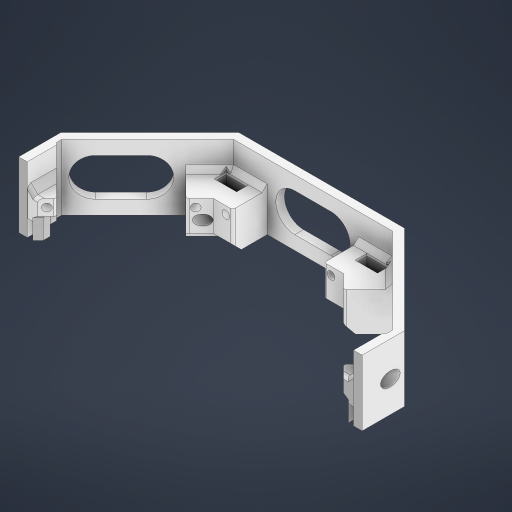
# Autodesk Inventor part: Držák TF-Luna
Saved by Autodesk Inventor 2024 (Build 280153000, 153)
## iProperties
Created: 2023-11-02
Part Number: Držák TF-Luna
Material: Všeobecné
Document SubType Name: Modeling
Designer: 42060
Density: 1 g/cm^3
Appearance: Výchozí
Author: 42060
Autodesk Inventor part; units mm, degrees
ref_plane "YZ Plane" through (0, 0, 0) normal (1, 0, 0) x (0, 1, 0)
ref_plane "XZ Plane" through (0, 0, 0) normal (0, 1, 0) x (-1, 0, 0)
ref_plane "XY Plane" through (0, 0, 0) normal (0, 0, 1) x (1, 0, 0)
sketch "Náčrt1" plane through (0, 0, 0) normal (0, 0, 1) x (1, 0, 0)
  line L0 (0, 0) -> (0, -2.5)
  line L1 (0, -2.5) -> (23, -2.5)
  line L2 (23, -2.5) -> (47.25, -26.75)
  line L3 (49.75, -25.714466) -> (24.035534, 0)
  line L4 (24.035534, 0) -> (0, 0)
  line L5 (49.75, -25.714466) -> (49.75, -37.923)
  line L6 (49.75, -37.923) -> (47.25, -37.923)
  line L7 (47.25, -37.923) -> (47.25, -26.75)
  dimension "d0" = 2.5
  dimension "d1" = 23
  dimension "d2" = 135
  dimension "d50" = 49.75
  dimension "d54" = 2.5
  dimension "d55" = 2.5
  dimension "d156" = 37.923
  constraints: 16 end point, 3 perpendicular, 2 vertical, 1 parallel
  measures "d0" distance of L0.start L0.end
  measures "d1" distance of L0.end L1.end
  measures "d2" angle of L2 L1
  measures "d50" distance between parallel lines of L5 L0
  measures "d54" distance between parallel lines of L2 L3
  measures "d55" distance between parallel lines of L5 L7
  measures "d156" distance between parallel lines of L6 L4
extrude "Vysunutí1" add sketch "Náčrt1" along normal mid plane 19
sketch "Náčrt2" plane through (0, -2.5, 9.5) normal (0, -1, 0) x (1, 0, 0)
  line L0 (23, -19) -> (23, 0) projected
  line L1 (0, 0) -> (23, 0) projected
  line L2 (0, -19) -> (0, 0) projected
  line L3 (23, -19) -> (0, -19) projected
  line L4 (13.25, -7.75) -> (15.25, -7.75)
  arc A0 (15.25, -12.25) -> (15.25, -7.75) centre (15.25, -10) ccw
  line L5 (15.25, -12.25) -> (13.25, -12.25)
  line L6 (13.25, -12.25) -> (13.25, -7.75)
  point P0 (0, -9.5)
  dimension "d6" = 2.25
  dimension "d8" = 9
  dimension "d148" = 13.25
  dimension "d149" = 15.25
  constraints: 6 end point, 2 point on circle, 2 tangent, 1 centre point, 1 horizontal, 1 parallel, 1 perpendicular
  measures "d6" radius of A0
  measures "d8" distance from line of L3 A0.centre
  measures "d148" distance between parallel lines of L6 L2
  measures "d149" distance from line of L2 A0.centre
extrude "Vysunutí2" add sketch "Náčrt2" along normal blind 10 contours L4 A0 L5 L6
sketch "Náčrt4" plane through (47.25, -26.75, 9.5) normal (-0.7071068, -0.7071068, 0) x (-0.7071068, 0.7071068, 0)
  line L0 (24.544679, 7.75) -> (26.544679, 7.75)
  arc A0 (26.544679, 7.75) -> (26.544679, 12.25) centre (26.544679, 10) ccw
  line L1 (26.544679, 12.25) -> (24.544679, 12.25)
  line L2 (24.544679, 12.25) -> (24.544679, 7.75)
  line L3 (0, 19) -> (0, 0)
  line L4 (34.294679, 0) -> (0, 0)
  line L5 (34.294679, 19) -> (34.294679, 0)
  line L6 (0, 19) -> (34.294679, 19)
  line L7 (41.18897, 12.25) -> (41.18897, 7.75)
  line L8 (11.294679, 19) -> (11.294679, 0) construction
  line L9 (-1.955321, 12.25) -> (-1.955321, 7.75)
  line L10 (-1.955321, 7.75) -> (-6.455321, 7.75)
  line L11 (-6.455321, 7.75) -> (-6.455321, 12.25)
  line L12 (-6.455321, 12.25) -> (-1.955321, 12.25)
  point P0 (52.325902, 9.5)
  point P1 (28.794679, 10)
  point P2 (-3.955321, 10)
  dimension "d22" = 15.25
  dimension "d33" = 2.25
  dimension "d39" = 5.5
  dimension "d150" = 13.25
  constraints: 16 end point, 4 perpendicular, 3 point on circle, 3 symmetric about line, 2 horizontal, 2 point on line, 2 tangent, 1 centre point, 1 horizontal alignment, 1 parallel, 1 vertical
  measures "d22" distance from line of L8 A0.centre
  measures "d33" radius of A0
  measures "d39" distance from line of L5 point (28.795, 10)
  measures "d150" distance between parallel lines of L8 L2
extrude "Vysunutí3" add sketch "Náčrt4" along normal blind 10 contours L2 L1 A0 L0 | L9 L10 L11 L12
sketch "Náčrt8" plane through (49.75, -37.923, 9.5) normal (1, 0, 0) x (0, 0, -1)
  line L0 (7.75, 8.673) -> (12.25, 8.673)
  line L1 (7.75, 6.608399) -> (7.75, 8.673)
  line L2 (12.25, 6.608399) -> (7.75, 6.608399)
  line L3 (12.25, 8.673) -> (12.25, 6.608399)
  line L4 (12.25, 4.543797) -> (7.75, 4.543797)
  line L5 (12.25, 6.608399) -> (12.25, 4.543797)
  line L6 (12.25, 6.608399) -> (7.75, 6.608399)
  line L7 (7.75, 6.608399) -> (7.75, 4.543797)
  point P0 (9.5, 37.923)
extrude "Vysunutí7" cut sketch "Náčrt8" along normal through all
sketch "Náčrt10" plane through (13.25, -2.5, 1.75) normal (0, 0, 1) x (1, 0, 0)
  line L0 (2, -10) -> (0, -10)
  line L1 (2, -10) -> (4.25, -10)
  line L2 (6.568019, -10.960155) -> (8.15901, -12.551145)
  line L3 (9.573223, -13.965359) -> (8.15901, -12.551145)
  line L4 (4.25, -10) -> (5.607864, -10)
  line L5 (5.607864, -10) -> (6.568019, -10.960155)
  circle A0 centre (7.844431, -4.600449) radius 3.594431
  line L6 (4.25, 0) -> (4.25, -10)
  line L7 (13.639087, -3.889087) -> (6.568019, -10.960155)
  line L8 (4.25, -4.600449) -> (2, -4.600449)
  line L9 (2, 0) -> (2, -10)
  line L10 (10.386078, -7.142096) -> (11.977069, -8.733087)
  line L11 (15.230078, -5.480078) -> (8.15901, -12.551145)
  line L12 (5.607864, -10) -> (6.468902, -7.921271) construction
  line L13 (-13.25, 0) -> (9.75, 0)
  line L14 (9.75, 0) -> (34, -24.25)
  point P0 (-13.25, 2.5)
  dimension "d70" = 112.5
  constraints: 10 end point, 4 point on line, 3 point on circle, 2 horizontal, 2 tangent, 1 centre point, 1 collinear, 1 equal length, 1 perpendicular
  measures "d70" angle of L4 L12
extrude "Vysunutí9" add sketch "Náčrt10" against normal up to surface (4.5 mm away) contours L9 L8 L6 L1 | L6 A0 L7 L5 L4 | L9 L13 L6 L8 | L7 L10 L11 L2 | L7 L14 L11 L10
sketch "Náčrt6" plane through (47.25, -26.75, 9.5) normal (-0.7071068, -0.7071068, 0) x (-0.7071068, 0.7071068, 0)
  arc A0 (11.391901, 8.259484) -> (11.391901, 10.740516) centre (16.544679, 9.5) ccw
  arc A1 (11.197457, 10.740516) -> (11.197457, 8.259484) centre (6.044679, 9.5) ccw
  line L0 (0, 19) -> (0, 0)
  line L1 (24.544679, 12.25) -> (24.544679, 7.75)
  line L2 (-1.955321, 7.75) -> (-1.955321, 12.25)
  line L3 (16.544679, 9.5) -> (24.544679, 9.5) construction
  line L4 (6.044679, 9.5) -> (-1.955321, 9.5) construction
  arc A2 (11.391901, 8.259484) -> (11.197457, 8.259484) centre (11.294679, 8.236078) ccw
  arc A3 (11.197457, 10.740516) -> (11.391901, 10.740516) centre (11.294679, 10.763922) ccw
  arc A4 (11.294679, 7.86064) -> (11.294679, 11.13936) centre (16.544679, 9.5) ccw
  arc A5 (11.294679, 11.13936) -> (11.294679, 7.86064) centre (6.044679, 9.5) ccw
  line L5 (16.544679, 4) -> (6.044679, 4)
  line L6 (16.544679, 15) -> (6.044679, 15)
  point P0 (52.325902, 9.5)
  point P1 (12.501786, 10.226292)
  point P2 (12.501786, 8.773708)
  point P3 (0, 9.5)
  point P4 (12.599008, 10.740516)
  point P5 (12.404563, 10.740516)
  point P6 (12.404563, 8.259484)
  point P7 (12.599008, 8.259484)
  dimension "d44" = 10.6
  dimension "d45" = 10.5
  dimension "d48" = 0.2
  dimension "d114" = 0.2
  constraints: 16 point on circle, 8 end point, 7 tangent, 6 centre point, 3 point on line, 2 equal radius, 2 horizontal alignment, 1 collinear, 1 midpoint, 1 parallel, 1 perpendicular, 1 other
  measures "d44" diameter of A1
  measures "d45" distance of L4.start L3.start
  measures "d48" diameter of A2
  measures "d114" radial gap between concentric circles of A0 A4
extrude "Vysunutí5" cut sketch "Náčrt6" against normal blind 11.5 contours A2 A1 A3 A0 | A5 A4 | A4 L5 A5 | A4 A5 L6
sketch "Náčrt7" plane through (0, -2.5, 9.5) normal (0, -1, 0) x (1, 0, 0)
  arc A0 (0.097222, -10.740516) -> (0.097222, -8.259484) centre (5.25, -9.5) ccw
  line L0 (0, -19) -> (0, 0)
  arc A1 (0, -8.336078) -> (0.097222, -8.259484) centre (0, -8.236078) ccw
  arc A2 (0.097222, -10.740516) -> (0, -10.663922) centre (0, -10.763922) ccw
  arc A3 (-0.097222, -8.259484) -> (-0.097222, -10.740516) centre (-5.25, -9.5) ccw
  arc A4 (-0.097222, -8.259484) -> (0, -8.336078) centre (0, -8.236078) ccw
  arc A5 (0, -10.663922) -> (-0.097222, -10.740516) centre (0, -10.763922) ccw
  arc A6 (0, -7.86064) -> (0, -11.13936) centre (-5.25, -9.5) ccw
  arc A7 (0, -11.13936) -> (0, -7.86064) centre (5.25, -9.5) ccw
  line L1 (-5.25, -4) -> (5.25, -4)
  line L2 (-5.25, -15) -> (5.25, -15)
  point P0 (0, -9.5)
  point P1 (0, -9.5)
  point P2 (0, -8.773708)
  point P3 (0, -10.226292)
  point P4 (0, -9.5)
  point P5 (0.097222, -8.259484)
  point P6 (0, -8.336078)
  point P7 (0, -10.663922)
  point P8 (0.097222, -10.740516)
  point P9 (0, -8.136078)
  point P10 (0, -10.863922)
  point P11 (0, -11.13936)
  point P12 (0, -15)
  point P13 (0, -4)
  dimension "d40" = 10.6
  dimension "d41" = 5.25
  dimension "d49" = 0.2
  dimension "d115" = 0.2
  constraints: 20 point on circle, 8 centre point, 6 tangent, 4 end point, 3 symmetric about line, 2 midpoint, 2 point on line, 2 vertical alignment, 1 equal radius, 1 horizontal alignment, 4 other
  measures "d40" diameter of A0
  measures "d41" distance from line of A0.centre L0
  measures "d49" diameter of A1
  measures "d115" radial gap between concentric circles of A3 A6
extrude "Vysunutí4" cut sketch "Náčrt7" against normal blind 11.5 contours A2 L0 A1 A0 | A0 A1 L0 A7 A2 | A5 A3 A4 L0 | A7 L2 L0 | L0 L1 A7
sketch "Náčrt11" plane through (0, 0, -9.5) normal (0, 0, -1) x (-1, 0, 0)
  line L0 (-23, -2.5) -> (0, -2.5)
  line L1 (-47.25, -26.75) -> (-23, -2.5)
  line L2 (-13.25, -2.5) -> (-13.25, -12.5)
  line L3 (-13.25, -12.5) -> (-18.857864, -12.5)
  line L4 (-18.857864, -12.5) -> (-22.823223, -16.465359)
  line L5 (-29.894291, -9.394291) -> (-22.823223, -16.465359)
  arc A0 (-23.636078, -9.642096) -> (-17.5, -7.100449) centre (-21.094431, -7.100449) ccw
  line L6 (-17.5, -7.100449) -> (-17.5, -2.5)
  line L7 (-26.889087, -6.389087) -> (-23.636078, -9.642096)
  point P0 (0, 0)
extrude "Vysunutí10" add sketch "Náčrt11" against normal up to surface (6.75 mm away) contours L0 L2 L3 L4 L5 L1 L7 A0 L6
sketch "Náčrt3" plane through (0, -12.5, 9.5) normal (0, -1, 0) x (1, 0, 0)
  arc A0 (15.25, -12.25) -> (15.25, -7.75) centre (15.25, -10) ccw projected
  point P0 (0, -9.5)
  constraints: 1 coincident
hole "Díra1" at (15.25, -12.5, -0.5) direction (0, 1, 0) diameter 2.2 end through all
sketch "Náčrt5" plane through (40.178932, -33.821068, 9.5) normal (-0.7071068, -0.7071068, 0) x (0, 0, -1)
  arc A0 (7.75, -26.544679) -> (12.25, -26.544679) centre (10, -26.544679) ccw
  line L0 (12.25, 6.455321) -> (7.75, 6.455321)
  line L1 (7.75, 6.455321) -> (7.75, 1.955321)
  line L2 (7.75, 1.955321) -> (12.25, 1.955321)
  line L3 (12.25, 1.955321) -> (12.25, 6.455321)
  line L4 (12.25, 1.955321) -> (12.25, 6.455321)
  line L5 (12.25, 6.455321) -> (7.75, 6.455321)
  line L6 (19, 1.035534) -> (0, 1.035534)
  line L7 (0, 9.668271) -> (0, 1.035534)
  line L8 (19, 9.668271) -> (0, 9.668271)
  line L9 (19, 1.035534) -> (19, 9.668271)
  line L10 (19, -11.294679) -> (0, -11.294679) construction
  point P0 (9.5, -52.325902)
  point P1 (10, 3.955321)
  constraints: 1 coincident, 1 symmetric about line
hole "Díra2" at (21.40901, -15.051145, -0.5) at (42.975767, -36.617902, -0.5) direction (0.7071068, 0.7071068, 0) diameter 2.2 end through all
chamfer "Zkosení3" [suppressed]
sketch "Náčrt9" plane through (47.25, -35.879203, 1.75) normal (0, 0, 1) x (1, 0, 0)
  line L0 (0, -2.043797) -> (0, 9.129203)
  line L1 (0, 0) -> (-2.506466, -2.506466)
  line L2 (0, -2.043797) -> (-2.043797, -2.043797)
  line L3 (-2.043797, -2.043797) -> (-2.969136, -2.043797)
  line L4 (-2.506466, -2.506466) -> (-5.688447, 0.675514)
  line L5 (0, 9.129203) -> (0, -2.043797)
  point P0 (-47.25, 35.879203)
  constraints: 4 end point, 2 horizontal, 2 point on line
extrude "Vysunutí8" add sketch "Náčrt9" against normal up to surface (4.5 mm away) contours L2 L1 L0
extrude "Vysunutí17" cut sketch "Náčrt9" against normal through all contours L1 L4 L3
sketch "Náčrt25" plane through (47.25, -35.879203, -2.75) normal (0, 0, -1) x (-1, 0, 0)
  line L0 (1.5, 2.956203) -> (1.5, -2.043797)
  line L1 (1.5, -2.043797) -> (3, -0.543797)
  line L2 (3, -0.543797) -> (3, 1.456203)
  line L3 (3, 1.456203) -> (1.5, 2.956203)
  line L4 (0, -2.043797) -> (0, 9.129203)
  point P0 (47.25, 35.879203)
  dimension "d185" = 45
  dimension "d188" = 1.5
  dimension "d189" = 5
  dimension "d190" = 1.5
  dimension "d191" = 45
  constraints: 8 end point, 1 horizontal alignment, 1 parallel, 1 vertical
  measures "d185" angle of L3 L0
  measures "d188" distance between parallel lines of L0 L2
  measures "d189" distance of L0.start L0.end
  measures "d190" distance between parallel lines of L4 L0
  measures "d191" angle of L0 L1
extrude "Vysunutí24" add sketch "Náčrt25" along normal up to surface (6.75 mm away)
chamfer "Zkosení4" [suppressed]
chamfer "Zkosení10" distance 2 angle 45 2 edges at (47.25, -33.7191, 1.75) (47.25, -33.7191, -2.75)
chamfer "Zkosení11" distance 1.0388 angle 45 3 edges at (44.75, -33.923, -2.75) (44.25, -35.423, -2.75) (44.75, -36.923, -2.75)
sketch "Náčrt26" plane through (47.25, -37.923, 9.5) normal (0, -1, 0) x (1, 0, 0)
  line L0 (0, -14.25) -> (-1.5, -14.25)
  line L1 (2.5, -19) -> (2.5, 0)
  line L2 (0, 0) -> (2.5, 0)
  line L3 (0, -5.75) -> (0, 0)
  line L4 (-2, -7.75) -> (0, -5.75)
  line L5 (-2.969136, -7.75) -> (-2, -7.75)
  line L6 (-2.969136, -12.25) -> (-2.969136, -7.75)
  line L7 (-2.969085, -12.25) -> (-2.969136, -12.25)
  line L8 (-2.969085, -12.25) -> (-1.5, -13.2888)
  line L9 (-1.5, -12.75) -> (-1.5, -13.2888)
  line L10 (0, -14.25) -> (-1.5, -12.75)
  line L11 (0, -19) -> (0, -14.25)
  line L12 (2.5, -19) -> (0, -19)
  line L13 (-1.5, -13.2888) -> (-1.5, -19)
  point P0 (-47.25, -9.5)
  constraints: 2 end point, 1 horizontal
extrude "Vysunutí25" add sketch "Náčrt26" against normal up to surface contours L0 L13 L9 L10 surface through (44.25, -34.423, -2.75) normal (-0.7071068, 0.7071068, 0)
extrude "Vysunutí21" add sketch "Náčrt11" against normal blind 2.5 contours L0 L6 A0 L7 L1
sketch "Náčrt22" plane through (17.5, -2.5, -7) normal (0, 0, 1) x (1, 0, 0)
  line L0 (0, -1.850449) -> (5.8, -1.850449)
  line L1 (5.8, -1.850449) -> (5.8, -4.600449)
  line L2 (5.8, -4.600449) -> (0, -4.600449)
  line L3 (0, -4.600449) -> (0, -1.850449)
  line L4 (0, -4.600449) -> (0, 0)
  arc A0 (0, -4.600449) -> (6.136078, -7.142096) centre (3.594431, -4.600449) ccw
  line L5 (9.389087, -3.889087) -> (6.136078, -7.142096)
  line L6 (5.5, 0) -> (9.389087, -3.889087)
  line L7 (0, 0) -> (5.5, 0)
  point P0 (-17.5, 2.5)
  point P1 (0, -1.850449)
  dimension "d163" = 5.8
  dimension "d164" = 2.75
  constraints: 8 end point, 2 parallel, 1 collinear, 1 horizontal, 1 perpendicular, 1 point on line
  measures "d163" distance of L1.end L2.end
  measures "d164" distance of L0.end L1.end
extrude "Vysunutí20" add sketch "Náčrt22" along normal up to surface (8.75 mm away) contours L4 L7 L6 L5 A0 L2 L1 L0
sketch "Náčrt23" plane through (17.5, -4.350449, -7) normal (0, -1, 0) x (1, 0, 0)
  line L0 (5.8, 8.75) -> (0, 8.75)
  line L1 (0, 0) -> (0, 8.75)
  line L2 (5.8, 0) -> (0, 0)
  line L3 (5.8, 0) -> (5.8, 8.75)
  line L4 (0, 1.674316) -> (2.9, 0)
  line L5 (2.9, 0) -> (5.8, 1.674316)
  circle A0 centre (2.9, 3.348632) radius 2.9 construction
  point P0 (-17.5, 7)
  dimension "d169" = 120
  constraints: 4 end point, 3 tangent, 2 point on line, 1 centre point, 1 horizontal alignment, 1 midpoint
  measures "d169" angle of L5 L4
extrude "Vysunutí22" add sketch "Náčrt23" along normal up to surface (2.75 mm away) contours L3 L2 L5 | L4 L2 L1
hole "Díra6" at (20.4, -4.350449, -3.651368) direction (0, 1, 0) diameter 3 end through all both
sketch "Náčrt24" plane through (0, 0, -9.5) normal (0, 0, -1) x (-1, 0, 0)
  line L0 (0, 0) -> (-24.035534, 0)
  line L1 (-21.9, 0) -> (-18.9, 0)
  line L2 (-18.9, -4.350449) -> (-21.9, -4.350449)
  line L3 (-24.491911, -3) -> (-16.308089, -3)
  line L4 (-24.491911, -3) -> (-23.4, 0)
  line L5 (-16.308089, -3) -> (-17.4, 0)
  point P0 (-20.4, -3)
  point P1 (-20.4, -4.350449)
  dimension "d180" = 3
  dimension "d183" = 70
  dimension "d184" = 70
  dimension "d209" = 6
  constraints: 6 end point, 2 midpoint, 2 point on line, 1 vertical alignment
  measures "d180" distance between parallel lines of L0 L3
  measures "d183" angle of L0 L4
  measures "d184" angle of L0 L5
  measures "d209" distance of L4.end L5.end
extrude "Vysunutí23" cut sketch "Náčrt24" against normal blind 10
fillet "Zaoblení1" radius 1 2 edges at (46.25, -37.923, 2.75) (44.7654, -37.923, 1.75)
chamfer "Zkosení5" distance 1.5 angle 45 2 edges at (26.4471, -5.9471, 1.75) (18.125, -2.5, 1.75)
sketch "Náčrt12" plane through (0, 0, 9.5) normal (0, 1, 0) x (1, 0, 0)
  circle A0 centre (15.25, 10) radius 1.1
  line L0 (15.25, 12.424871) -> (17.35, 11.212436)
  line L1 (17.35, 11.212436) -> (17.35, 8.787564)
  line L2 (17.35, 8.787564) -> (15.25, 7.575129)
  line L3 (15.25, 7.575129) -> (13.15, 8.787564)
  line L4 (13.15, 8.787564) -> (13.15, 11.212436)
  line L5 (13.15, 11.212436) -> (15.25, 12.424871)
  point P0 (0, 9.5)
  point P1 (15.25, 10)
  dimension "d81" = 4.2
  constraints: 12 end point, 1 coincident, 1 vertical alignment, 13 other
  measures "d81" distance between parallel lines of L4 L1
extrude "Vysunutí12" [suppressed]
sketch "Náčrt13" plane through (24.035534, 0, -9.5) normal (0.7071068, 0.7071068, 0) x (-0.7071068, 0.7071068, 0)
  circle A0 centre (-8.785534, 9) radius 1.1
  line L0 (-8.785534, 6.575129) -> (-10.885534, 7.787564)
  line L1 (-10.885534, 7.787564) -> (-10.885534, 10.212436)
  line L2 (-10.885534, 10.212436) -> (-8.785534, 11.424871)
  line L3 (-8.785534, 11.424871) -> (-6.685534, 10.212436)
  line L4 (-6.685534, 10.212436) -> (-6.685534, 7.787564)
  line L5 (-6.685534, 7.787564) -> (-8.785534, 6.575129)
  line L6 (-39.285534, 6.575129) -> (-41.385534, 7.787564)
  line L7 (-41.385534, 7.787564) -> (-41.385534, 10.212436)
  line L8 (-41.385534, 10.212436) -> (-39.285534, 11.424871)
  line L9 (-39.285534, 11.424871) -> (-37.185534, 10.212436)
  line L10 (-37.185534, 10.212436) -> (-37.185534, 7.787564)
  line L11 (-37.185534, 7.787564) -> (-39.285534, 6.575129)
  circle A1 centre (-39.285534, 9) radius 1.1
  point P0 (16.995689, 9.5)
  point P1 (-39.285534, 9)
  point P2 (-39.285534, 9)
  dimension "d84" = 4.2
  dimension "d85" = 4.2
  constraints: 24 end point, 3 coincident, 1 vertical alignment, 26 other
  measures "d84" distance between parallel lines of L4 L1
  measures "d85" distance between parallel lines of L7 L10
extrude "Vysunutí13" [suppressed]
extrude "Vysunutí14" [suppressed]
sketch "Náčrt15" plane through (0, 0, 9.5) normal (0, 1, 0) x (1, 0, 0)
  circle A0 centre (15.25, 10) radius 1.1 projected
  point P0 (0, 9.5)
  point P1 (15.25, 10)
  constraints: 1 coincident
hole "Díra3" at (15.25, 0, -0.5) direction (0, -1, 0) diameter 4 depth 2
sketch "Náčrt16" plane through (24.035534, 0, -9.5) normal (0.7071068, 0.7071068, 0) x (-0.7071068, 0.7071068, 0)
  circle A0 centre (-8.785534, 9) radius 1.1
  point P0 (16.995689, 9.5)
  constraints: 1 coincident
hole "Díra4" at (30.247845, -6.212311, -0.5) direction (-0.7071068, -0.7071068, 0) diameter 4 depth 2
sketch "Náčrt17" plane through (24.035534, 0, -9.5) normal (0.7071068, 0.7071068, 0) x (-0.7071068, 0.7071068, 0)
  circle A0 centre (-39.285534, 9) radius 1.1
  point P0 (16.995689, 9.5)
  point P1 (-39.285534, 9)
  point P2 (-39.285534, 9)
  constraints: 2 coincident
hole "Díra5" at (51.814601, -27.779067, -0.5) direction (-0.7071068, -0.7071068, 0) diameter 4 depth 6
sketch "Náčrt14" plane through (49.75, -37.923, 9.5) normal (1, 0, 0) x (0, 0, -1)
  line L0 (19, 12.208534) -> (0, 12.208534)
  line L1 (19, 12.208534) -> (23, 12.208534)
  line L2 (23, 12.208534) -> (23, 6.208534)
  line L3 (23, 6.208534) -> (21, 6.208534)
  line L4 (21, 6.208534) -> (21, 10.208534)
  line L5 (21, 10.208534) -> (19, 10.208534)
  line L6 (19, 12.208534) -> (19, 0)
  point P0 (9.5, 37.923)
  point P1 (11.381206, 11.708534)
  dimension "d105" = 2
  dimension "d106" = 2
  dimension "d107" = 6
  dimension "d108" = 4
  constraints: 10 end point, 3 perpendicular, 1 horizontal, 1 vertical, 1 other
  measures "d105" distance between parallel lines of L1 L5
  measures "d106" distance between parallel lines of L4 L2
  measures "d107" distance between parallel lines of L1 L3
  measures "d108" distance between parallel lines of L6 L2
extrude "Vysunutí15" [suppressed]
chamfer "Zkosení7" [suppressed]
chamfer "Zkosení1" distance 2.5 angle 45 2 edges at (16.0539, -12.5, -9.5) (20.8405, -14.4827, -9.5)
fillet "Zaoblení3" radius 0.7 3 edges at (13.25, -12.5, -2.625) (22.8232, -16.4654, -2.625) (41.5616, -35.2037, -0.5)
sketch "Náčrt19" plane through (49.75, -37.923, 9.5) normal (1, 0, 0) x (0, 0, -1)
  line L0 (0, 11.173) -> (0, 0) projected
  line L1 (0, 0) -> (19, 0)
  line L2 (19, 0) -> (19, -0.077)
  line L3 (19, -0.077) -> (0, -0.077)
  line L4 (0, -0.077) -> (0, 0)
  point P0 (9.5, 37.923)
  dimension "d153" = 38
  constraints: 8 end point, 2 parallel, 1 horizontal, 1 perpendicular
  measures "d153" distance from line of point (9.5, 37.923) L3
extrude "Vysunutí18" add sketch "Náčrt19" against normal up to surface (2.5 mm away)
sketch "Náčrt20" plane through (0, 0, 9.5) normal (0, 0, 1) x (1, 0, 0)
  line L0 (23, -2.5) -> (47.25, -26.75)
  line L1 (47.25, -26.75) -> (48.632621, -28.132621)
  line L2 (48.632621, -28.132621) -> (47.25, -29.515242)
  line L3 (47.25, -26.75) -> (47.25, -38)
  line L4 (47.882621, -27.382621) -> (47.882621, -28.882621)
  line L5 (45.25, -31.515242) -> (42.056528, -34.708714)
  point P0 (0, 0)
  dimension "d159" = 0.75
  constraints: 6 end point, 4 point on line, 1 collinear, 1 perpendicular, 1 vertical
  measures "d159" distance from line of L1.end L4
extrude "Vysunutí19" cut sketch "Náčrt20" against normal through all contours L1 L4 L2 L3
chamfer "Zkosení12" distance 0.75 angle 45 1 edges at (46.5, -32.173, -4)
chamfer "Zkosení13" distance 0.35 angle 45 4 edges at (20.4, -7.1004, 1.75) (20.1146, -4.3504, 1.75) (23.3, -6.0109, 1.75) (17.5, -5.7254, 1.75)
ref_plane "Pracovní rovina1" through (23.3, -4.350449, -5.325684) normal (0.7071068, -0.7071068, 0) x (0, 0, 1)
sketch "Náčrt29" plane through (17.5, -7.100449, 1.4) normal (0, 1, 0) x (1, 0, 0)
  line L0 (5.8, -0.7) -> (5.8, -0.753667)
  line L1 (5.8, 0) -> (5.8, -0.753667)
  line L2 (6.15, -0.35) -> (11.333631, -0.35)
  line L3 (11.333631, -0.35) -> (12.394291, -1.85)
  line L4 (12.394291, -1.85) -> (5.5, -1.85)
  line L5 (4.87868, -0.35) -> (5.5, -1.85)
  line L6 (4.87868, -0.35) -> (4.879129, -0.35)
  line L7 (5.8, -0.753667) -> (4.734154, 0)
  line L8 (6.15, -0.35) -> (5.8, 0)
  line L9 (4.734154, 0) -> (4.879129, -0.35)
  line L10 (6.15, -0.35) -> (6.15, -1.85)
  point P0 (-17.5, 1.4)
  point P1 (6.45, -1.85)
  point P2 (5.8, -0.7)
  constraints: 2 end point, 2 point on line, 1 perpendicular
extrude "Vysunutí27" cut sketch "Náčrt29" against normal up to surface contours L1 L8 L10 L4 L5 L9 L7 L0 surface through (23.3, -4.350449, -5.325684) normal (0.7071068, -0.7071068, 0)
sketch "Náčrt30" plane through (17.5, -7.100449, -5.325684) normal (1, 0, 0) x (0, 0, -1)
  line L0 (-7.479351, 2.75) -> (-7.974326, 3.1)
  line L1 (-7.075684, 1.829129) -> (-7.075684, -3.354502)
  line L2 (-7.075684, -3.354502) -> (-8.575684, -2.293842)
  line L3 (-7.075684, 3.100449) -> (-8.575684, 4.600449)
  line L4 (-7.075684, 3.100449) -> (-7.075684, 3.1)
  line L5 (-7.479351, 2.75) -> (-6.725684, 2.75)
  line L6 (-8.575684, -2.293842) -> (-8.575684, 4.600449)
  line L7 (-6.725684, 2.75) -> (-7.075684, 3.1)
  line L8 (-7.974326, 3.1) -> (-7.075684, 1.829129)
  line L9 (-7.075684, 1.829129) -> (-7.075684, 3.1)
  line L10 (-7.974326, 3.1) -> (-7.075684, 3.1)
  point P0 (-5.325684, 7.100449)
extrude "Vysunutí28" cut sketch "Náčrt30" along normal up to surface contours L0 L10 L9 L5 | L9 L7 L5 surface through (23.3, -4.350449, -5.325684) normal (0.7071068, -0.7071068, 0)
chamfer "Zkosení14" distance 0.25 angle 45 2 edges at (23.0146, -4.0004, 2.1993) (23.65, -4.6359, 2.1993)
mirror "Zrcadlit1" about plane through (0, 0, 0) normal (1, 0, 0)
